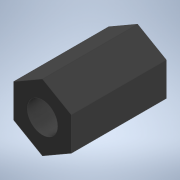
# Autodesk Inventor part: Separadores_PCB
Saved by Autodesk Inventor 2020 (Build 240168000, 168)
## iProperties
Created: 2020-08-08
Part Number: Separadores_PCB
Material: Generic
Document SubType Name: Modeling
Designer: Erick Miranda
Density: 1 g/cm^3
Appearance: Default
Author: Erick Miranda
Autodesk Inventor part; units mm, degrees
ref_plane "YZ Plane" through (0, 0, 0) normal (1, 0, 0) x (0, 1, 0)
ref_plane "XZ Plane" through (0, 0, 0) normal (0, 1, 0) x (-1, 0, 0)
ref_plane "XY Plane" through (0, 0, 0) normal (0, 0, 1) x (1, 0, 0)
sketch "Sketch1" plane through (0, 0, 0) normal (0, 0, 1) x (1, 0, 0)
  circle A0 centre (0, 0) radius 1.6
  line L0 (0, 0) -> (0, 3.5)
  line L1 (0, 3.5) -> (3.0311, 1.75)
  line L2 (3.0311, 1.75) -> (3.0311, -1.75)
  line L3 (3.0311, -1.75) -> (0, -3.5)
  line L4 (0, -3.5) -> (-3.0311, -1.75)
  line L5 (-3.0311, -1.75) -> (-3.0311, 1.75)
  line L6 (-3.0311, 1.75) -> (0, 3.5)
  dimension "d0" = 3.2
  dimension "d1" = 3.5
  constraints: 14 end point, 2 coincident, 1 centre point, 1 vertical, 13 other
  measures "d0" diameter of A0
  measures "d1" distance of L0.start L0.end
extrude "Extrusion1" add sketch "Sketch1" along normal blind 10
body "Solid1"
